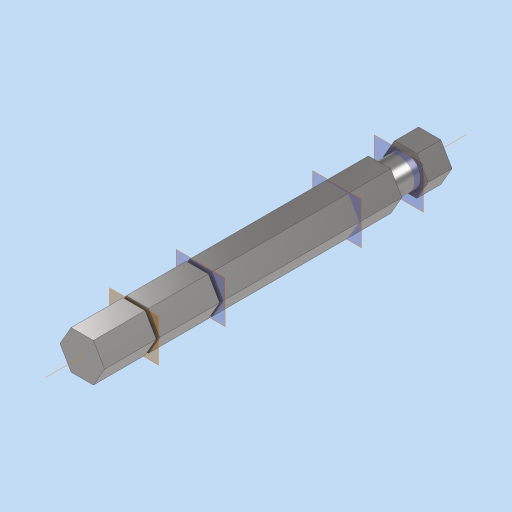
# Autodesk Inventor part: Ch-1-01-0.5x4.5HexShaft
Saved by Autodesk Inventor 2024 (Build 280153000, 153)
## iProperties
Created: 2022-11-08
Part Number: Ch-1-01-0.5x4.5HexShaft
Material: Steel, Alloy
Document SubType Name: Modeling
Designer: megan
Density: 7.73 g/cm^3
Appearance: Semi-Polished
Author: megan
Autodesk Inventor part; units mm, degrees
ref_plane "YZ Plane" through (0, 0, 0) normal (1, 0, 0) x (0, 1, 0)
ref_plane "XZ Plane" through (0, 0, 0) normal (0, 1, 0) x (-1, 0, 0)
ref_plane "XY Plane" through (0, 0, 0) normal (0, 0, 1) x (1, 0, 0)
sketch "Sketch1" plane through (0, 0, 0) normal (0, 0, 1) x (1, 0, 0)
  line L0 (7.3323, 0) -> (3.6662, -6.35)
  line L1 (3.6662, -6.35) -> (-3.6662, -6.35)
  line L2 (-3.6662, -6.35) -> (-7.3323, 0)
  line L3 (-7.3323, 0) -> (-3.6662, 6.35)
  line L4 (-3.6662, 6.35) -> (3.6662, 6.35)
  line L5 (3.6662, 6.35) -> (7.3323, 0)
  point P0 (0, 0)
  point P1 (0, 0)
  dimension "d0" = 12.7
  constraints: 12 end point, 1 coincident, 13 other
  measures "d0" distance between parallel lines of L5 L2
extrude "Extrusion1" add sketch "Sketch1" along normal mid plane 114.3
sketch "Sketch10" plane through (0, 0, -57.15) normal (0, 0, -1) x (-1, 0, 0)
  point P0 (0, 0)
  point P1 (0, 0)
  constraints: 1 coincident
hole "Hole3" at (0, 0, -57.15) direction (0, 0, 1) diameter 3.9624 depth 13.6144 tip angle 118 thread size "10-32 UNF" class "2B" standard "ANSI Unified Screw Threads"
ref_plane "Work Plane4" through (0, 0, -46.99) normal (0, 0, -1) x (-1, 0, 0)
ref_plane "Work Plane5" through (0, 0, -26.67) normal (0, 0, -1) x (-1, 0, 0)
ref_plane "Work Plane6" through (0, 0, 18.2372) normal (0, 0, -1) x (-1, 0, 0)
sketch "Sketch13" plane through (0, 0, 18.2372) normal (0, 0, -1) x (-1, 0, 0)
  circle A0 centre (0, 0) radius 1.9812
  circle A1 centre (0, 0) radius 4.9784
  line L0 (3.6662, -6.35) -> (7.3323, 0)
  circle A2 centre (0, 0) radius 7.3323
  dimension "d51" = 9.9568
  constraints: 2 centre point, 2 coincident, 2 end point, 1 horizontal alignment, 2 other
  measures "d51" diameter of A1
extrude "Extrusion7" cut sketch "Sketch13" against normal blind 1.0668 contours A2 L0 | L0 A2
ref_plane "Work Plane7" through (0, 0, 40.132) normal (0, 0, 1) x (1, 0, 0)
sketch "Sketch15" plane through (0, 0, 40.132) normal (0, 0, 1) x (1, 0, 0)
  circle A0 centre (0, 0) radius 1.9812
  circle A1 centre (0, 0) radius 4.9784
  line L0 (3.6662, -6.35) -> (7.3323, 0)
  circle A2 centre (0, 0) radius 7.3323
  dimension "d60" = 9.9568
  constraints: 2 centre point, 2 coincident, 2 end point, 1 horizontal alignment, 2 other
  measures "d60" diameter of A1
extrude "Extrusion9" cut sketch "Sketch15" against normal blind 1.0668 contours A2 L0 | L0 A2
sketch "Sketch16" plane through (0, 0, 39.0652) normal (0, 0, 1) x (1, 0, 0)
  point P0 (0, 0)
sketch "Sketch17" plane through (0, 0, -46.99) normal (0, 0, -1) x (-1, 0, 0)
  circle A0 centre (0, 0) radius 1.9812 projected
  circle A1 centre (0, 0) radius 5.08
  line L0 (-3.6662, 6.35) -> (3.6662, 6.35) projected
  line L1 (3.6662, 6.35) -> (7.3323, 0) projected
  line L2 (7.3323, 0) -> (3.6662, -6.35) projected
  line L3 (3.6662, -6.35) -> (-3.6662, -6.35) projected
  line L4 (-3.6662, -6.35) -> (-7.3323, 0) projected
  line L5 (-7.3323, 0) -> (-3.6662, 6.35) projected
  dimension "d64" = 10.16
  constraints: 1 centre point, 1 coincident
  measures "d64" diameter of A1
extrude "Extrusion10" cut sketch "Sketch17" along normal blind 2.2098 and the other way blind 6.35 contours L0 L1 L2 L3 L4 L5
body "Solid1"
